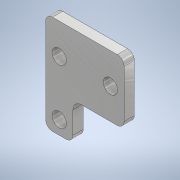
# Autodesk Inventor part: L_almite_braket
Saved by Autodesk Inventor 2022 (Build 260153000, 153)
## iProperties
Created: 2020-07-22
Part Number: L_almite_braket
Material: 一般
Document SubType Name: Sheet Metal
Designer: gisen
Density: 1 g/cm^3
Sheet Metal Rule: Default_mm
Appearance: 機械加工 - アルミニウム
Mass: 1.63791 g
Surface Area: 15.668 cm^2
Volume: 1.63791 cm^3
Author: gisen
Autodesk Inventor part; units mm, degrees
ref_plane "YZ Plane" through (0, 0, 0) normal (1, 0, 0) x (0, 1, 0)
ref_plane "XZ Plane" through (0, 0, 0) normal (0, 1, 0) x (-1, 0, 0)
ref_plane "XY Plane" through (0, 0, 0) normal (0, 0, 1) x (1, 0, 0)
sketch "スケッチ1" plane through (0, 0, 0) normal (0, 1, 0) x (-1, 0, 0)
  line L0 (-3, 9) -> (16, 9)
  line L1 (10, -9) -> (-3, -9)
  line L2 (-5, -7) -> (-5, 7)
  line L3 (16, -20) -> (12, -20)
  line L4 (10, -18) -> (10, -9)
  arc A0 (16, -20) -> (18, -18) centre (16, -18) ccw
  arc A1 (10, -18) -> (12, -20) centre (12, -18) ccw
  arc A2 (-5, -7) -> (-3, -9) centre (-3, -7) ccw
  arc A3 (-3, 9) -> (-5, 7) centre (-3, 7) ccw
  line L5 (18, 7) -> (18, -18)
  arc A4 (18, 7) -> (16, 9) centre (16, 7) ccw
  point P0 (0, 0)
  point P1 (-5, 9)
  point P2 (-5, -9)
  point P3 (18, -20)
  point P4 (10, -20)
  point P5 (10, 9)
  point P6 (18, 9)
  dimension "d0" = 5
  dimension "d4" = 18
  dimension "d5" = 9
  dimension "d7" = 20
  dimension "d8" = 10
  dimension "d40" = 2
  constraints: 12 end point, 10 point on circle, 10 point on line, 10 tangent, 5 centre point, 3 equal radius, 2 parallel, 1 horizontal, 1 perpendicular
  measures "d0" distance from line of L2 point (0, 0)
  measures "d4" distance between parallel lines of L0 L1
  measures "d5" distance from line of L0 point (0, 0)
  measures "d7" distance from line of point (0, 0) L3
  measures "d8" distance from line of point (0, 0) L4
  measures "d40" radius of A4
extrude "プレート1" add sketch "スケッチ1" along normal blind 3
sketch "スケッチ3" plane through (0, 3, 0) normal (0, 1, 0) x (1, 0, 0)
  line L0 (-10, 18) -> (-10, 9) projected
  line L1 (-16, 20) -> (-12, 20) projected
  line L2 (-18, -7) -> (-18, 18) projected
  line L3 (-10, 9) -> (3, 9) projected
  line L4 (3, -9) -> (-16, -9) projected
  point P0 (-14, 16)
  point P1 (-14, 0)
  dimension "d42" = 4
  dimension "d43" = 4
  dimension "d44" = 4
  dimension "d45" = 18
  dimension "d46" = 9
  measures "d42" distance from line of point (-14, 16) L1
  measures "d43" distance from line of point (-14, 16) L2
  measures "d44" distance from line of L2 point (-14, 0)
  measures "d45" distance between parallel lines of L3 L4
  measures "d46" distance from line of point (-14, 0) L4
hole "穴3" at (1, 3, 0) direction (0, -1, 0) diameter 4.2 end through all
sketch "スケッチ2" plane through (0, 0, 0) normal (0, -1, 0) x (1, 0, 0)
  circle A0 centre (1, 0) radius 2.1 projected
  line L0 (3, 9) -> (-16, 9) projected
  arc A1 (-18, -18) -> (-16, -20) centre (-16, -18) ccw projected
  line L1 (-16, -20) -> (-12, -20) projected
  arc A2 (-12, -20) -> (-10, -18) centre (-12, -18) ccw projected
  line L2 (-10, -18) -> (-10, -9) projected
  line L3 (-10, -9) -> (3, -9) projected
  arc A3 (3, -9) -> (5, -7) centre (3, -7) ccw projected
  line L4 (5, -7) -> (5, 7) projected
  arc A4 (5, 7) -> (3, 9) centre (3, 7) ccw projected
  line L5 (-18, 7) -> (-18, -18) projected
  arc A5 (-16, 9) -> (-18, 7) centre (-16, 7) ccw projected
  point P0 (0, 0)
fillet "フィレット1" radius 2.5 1 edges at (-10, 1.5, -9)
hole "穴4" at (-14, 3, -16) at (-14, 3, 0) direction (0, -1, 0) diameter 4.2 end through all
equation "\"d5\" = 0.5 * d4"
equation "\"d7\" = 0.5 * d6"
equation "\"d44\" = d43"
equation "\"d37\" = Thickness"
equation "\"d52\" = Thickness"
equation "\"d9\" = Thickness"
equation "\"BendRadius\" = Thickness"
equation "\"BendReliefWidth\" = Thickness"
equation "\"BendReliefDepth\" = 0.5 * Thickness"
equation "\"CornerReliefSize\" = 4 * Thickness"
equation "\"MinimumRemnant\" = 2 * Thickness"
equation "\"TransitionRadius\" = BendRadius"
equation "\"JacobiRadiusSize\" = BendRadius"
equation "\"GapSize\" = Thickness"
equation "\"Thickness\" = 3"
equation "\"d6\" = 40"
